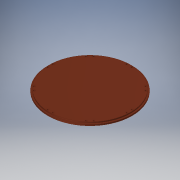
# Autodesk Inventor part: 4K sheild top
Saved by Autodesk Inventor 2018 (Build 220112000, 112)
## iProperties
Created: 2019-03-11
Part Number: 4K sheild top
Material: Copper
Document SubType Name: Modeling
Designer: Admin
Density: 8.94 g/cm^3
Appearance: Copper - Satin
Author: Admin
Autodesk Inventor part; units mm, degrees
ref_plane "YZ Plane" through (0, 0, 0) normal (1, 0, 0) x (0, 1, 0)
ref_plane "XZ Plane" through (0, 0, 0) normal (0, 1, 0) x (-1, 0, 0)
ref_plane "XY Plane" through (0, 0, 0) normal (0, 0, 1) x (1, 0, 0)
sketch "Sketch1" plane through (0, 0, 0) normal (0, 1, 0) x (-1, 0, 0)
  circle A0 centre (0, 0) radius 101.6
  dimension "d0" = 203.2
  constraints: 1 centre point, 1 coincident
  measures "d0" diameter of A0
extrude "Extrusion1" add sketch "Sketch1" along normal blind 6.35
sketch "Sketch3" plane through (0, 6.35, 0) normal (0, 1, 0) x (1, 0, 0)
  line L0 (0, 0) -> (67.3519, 67.3519) construction
  line L1 (0, 0) -> (95.25, 0) construction
  line L2 (67.3519, 67.3519) -> (71.842, 62.8618) construction
  point P0 (62.8618, 71.842)
  point P1 (62.8618, 71.842)
  dimension "d14" = 95.25
  dimension "d15" = 45
  dimension "d16" = 6.35
  dimension "d17" = 90
  constraints: 6 end point, 2 coincident, 1 equal length, 1 horizontal, 1 symmetric about line
  measures "d14" distance of L0.start L0.end
  measures "d15" angle of L1 L0
  measures "d16" distance of L0.end L2.end
  measures "d17" angle of L2 L0
hole "Hole2" at (71.842, 6.35, -62.8618) at (62.8618, 6.35, -71.842) direction (0, -1, 0) diameter 3.81 depth 8.8646 tip angle 118 clearance for "Flat Head Machine Screw (82)" size "#6" standard "Ansi Unified Screw Threads"
pattern_circular "Circular Pattern2" count 8 over 360 about axis through (0, 0, 0) along (0, 1, 0) of "Hole2"
sketch "Sketch4" plane through (0, 6.35, 0) normal (0, 1, 0) x (1, 0, 0)
  circle A0 centre (0, 0) radius 101.6
  circle A1 centre (0, 0) radius 101.6 projected
  circle A2 centre (0, 0) radius 98.425
  dimension "d28" = 196.85
  constraints: 2 centre point, 2 coincident, 2 concentric
  measures "d28" diameter of A2
extrude "Extrusion2" cut sketch "Sketch4" against normal blind 3.175
body "Solid1"
